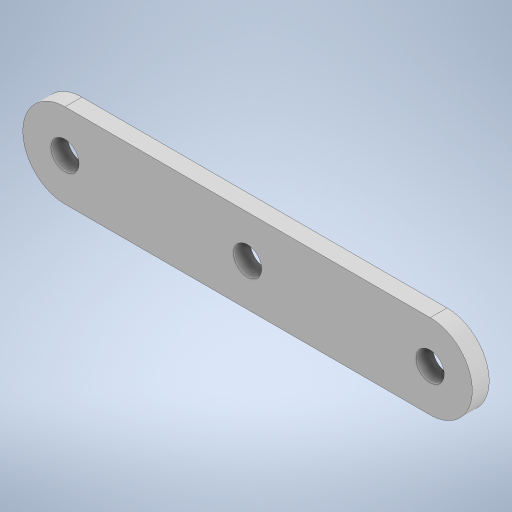
# Autodesk Inventor part: DP3_linkage_extruded
Saved by Autodesk Inventor 2024 (Build 280153000, 153)
## iProperties
Created: 2024-01-29
Part Number: DP3_linkage_extruded
Material: Generic
Document SubType Name: Modeling
Designer: clbri
Density: 1 g/cm^3
Appearance: Default
Author: clbri
Autodesk Inventor part; units mm, degrees
ref_plane "YZ Plane" through (0, 0, 0) normal (1, 0, 0) x (0, 1, 0)
ref_plane "XZ Plane" through (0, 0, 0) normal (0, 1, 0) x (-1, 0, 0)
ref_plane "XY Plane" through (0, 0, 0) normal (0, 0, 1) x (1, 0, 0)
sketch "Sketch1" plane through (0, 0, 0) normal (0, 0, 1) x (1, 0, 0)
  line L0 (7.5, 0) -> (72.5, 0)
  line L1 (72.5, 15) -> (7.5, 15)
  arc A0 (7.5, 15) -> (7.5, 0) centre (7.5, 7.5) ccw
  arc A1 (72.5, 0) -> (72.5, 15) centre (72.5, 7.5) ccw
  circle A2 centre (7.5, 7.5) radius 2.5
  circle A3 centre (72.5, 7.5) radius 2.5
  circle A4 centre (40, 7.5) radius 2.5
  point P0 (0, 0)
  point P1 (0, 7.5)
  point P2 (40, 15)
  dimension "d7" = 5
  dimension "d8" = 5
  dimension "d9" = 5
  dimension "d10" = 40
  dimension "d11" = 7.5
  constraints: 5 centre point, 5 point on circle, 4 end point, 2 coincident, 1 horizontal, 1 midpoint, 1 parallel
  measures "d7" diameter of A2
  measures "d8" diameter of A3
  measures "d9" diameter of A4
  measures "d10" distance of point (0, 7.5) A4.centre
  measures "d11" distance of point (40, 15) A4.centre
extrude "Extrusion1" add sketch "Sketch1" along normal blind 3
body "Solid1"
